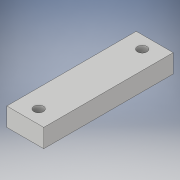
# Autodesk Inventor part: servo hold down
Saved by Autodesk Inventor 2018 (Build 220112000, 112)
## iProperties
Created: 2018-06-18
Part Number: servo hold down
Material: Generic
Document SubType Name: Sheet Metal
Designer: mmarkle
Density: 1 g/cm^3
Sheet Metal Rule: Default
Appearance: Default
Author: mmarkle
Autodesk Inventor part; units mm, degrees
ref_plane "YZ Plane" through (0, 0, 0) normal (1, 0, 0) x (0, 1, 0)
ref_plane "XZ Plane" through (0, 0, 0) normal (0, 1, 0) x (-1, 0, 0)
ref_plane "XY Plane" through (0, 0, 0) normal (0, 0, 1) x (1, 0, 0)
sketch "Sketch1" plane through (0, 0, 0) normal (0, 1, 0) x (-1, 0, 0)
  line L0 (-0.8262, 0) -> (11.8738, 0)
  line L1 (11.8738, 0) -> (11.8738, -44.45)
  line L2 (11.8738, -44.45) -> (-0.8262, -44.45)
  line L3 (-0.8262, -44.45) -> (-0.8262, 0)
  point P0 (0, 0)
  dimension "d0" = 44.45
  dimension "d1" = 12.7
  measures "d0" distance of L2.end L0.start
  measures "d1" distance of L0.start L0.end
extrude "Plate1" add sketch "Sketch1" along normal blind 6.35
sketch "Sketch2" plane through (0, 6.35, 0) normal (0, 1, 0) x (1, 0, 0)
  line L0 (0.8262, 0) -> (-11.8738, 0) projected
  line L1 (0.8262, 44.45) -> (0.8262, 0) projected
  point P0 (0, 0)
  point P1 (-5.5238, 4.5974)
  point P2 (-5.5238, 40.1574)
  dimension "d4" = 35.56
  dimension "d5" = 4.5974
  dimension "d6" = 6.35
  dimension "d7" = 6.35
  measures "d4" distance of point (-5.524, 40.157) point (-5.524, 4.597)
  measures "d5" distance from line of L0 point (-5.524, 4.597)
  measures "d6" distance from line of L1 point (-5.524, 40.157)
  measures "d7" distance from line of L1 point (-5.524, 4.597)
hole "Hole1" at (-5.5238, 6.35, -4.5974) at (-5.5238, 6.35, -40.1574) direction (0, -1, 0) diameter 3.2766 end through all clearance for "Flat Head Machine Screw (82)" size "#4" standard "Ansi Unified Screw Threads"
equation "\"d13\" = Thickness"
equation "\"d2\" = Thickness"
equation "\"BendRadius\" = Thickness"
equation "\"BendReliefWidth\" = Thickness"
equation "\"BendReliefDepth\" = 0.5 * Thickness"
equation "\"CornerReliefSize\" = 4 * Thickness"
equation "\"MinimumRemnant\" = 2 * Thickness"
equation "\"TransitionRadius\" = BendRadius"
equation "\"JacobiRadiusSize\" = BendRadius"
equation "\"GapSize\" = Thickness"
equation "\"Thickness\" = 6.35"
body "Solid1"
